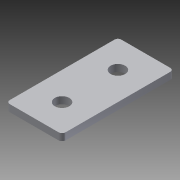
# Autodesk Inventor part: Chassis Connector Plate V1.500
Saved by Autodesk Inventor 2014 SP1 (Build 180222100, 222)
## iProperties
Created: 2013-01-14
Part Number: Chassis Connector Plate V1.500
Material: Aluminum 6061
Document SubType Name: Modeling
Designer: Moses
Density: 2.71 g/cm^3
Mass: 10.4942 g
Surface Area: 30.4626 cm^2
Volume: 3.87239 cm^3
Appearance: Aluminum - Flat
Author: Moses
Autodesk Inventor part; units mm, degrees
ref_plane "YZ Plane" through (0, 0, 0) normal (1, 0, 0) x (0, 1, 0)
ref_plane "XZ Plane" through (0, 0, 0) normal (0, 1, 0) x (-1, 0, 0)
ref_plane "XY Plane" through (0, 0, 0) normal (0, 0, 1) x (1, 0, 0)
sketch "Sketch1" plane through (0, 0, 0) normal (0, 1, 0) x (-1, 0, 0)
  line L0 (0, 0) -> (0, 50.8)
  line L1 (0, 50.8) -> (25.4, 50.8)
  line L2 (25.4, 50.8) -> (25.4, 0)
  line L3 (25.4, 0) -> (0, 0)
  circle A0 centre (12.7, 38.1) radius 3.302
  circle A1 centre (12.7, 12.7) radius 3.302
  line L4 (0, 25.4) -> (25.4, 25.4) construction
  line L5 (12.7, 38.1) -> (12.7, 12.7) construction
  point P0 (12.7, 25.4)
  dimension "d0" = 50.8
  dimension "d1" = 25.4
  dimension "d2" = 6.604
  dimension "d3" = 6.604
  dimension "d4" = 25.4
  constraints: 12 end point, 4 midpoint, 2 centre point, 2 parallel, 2 perpendicular, 1 vertical
  measures "d0" distance of L0.start L0.end
  measures "d1" distance of L0.end L1.end
  measures "d2" diameter of A0
  measures "d3" diameter of A1
  measures "d4" distance of L5.start L5.end
extrude "Extrusion1" add sketch "Sketch1" along normal blind 3.175
fillet "Fillet1" radius 1.5875 4 edges at (-25.4, 1.5875, 50.8) (0, 1.5875, 50.8) (0, 1.5875, 0) (-25.4, 1.5875, 0)
equation "\"d3\" = d2"
body "Solid1"
